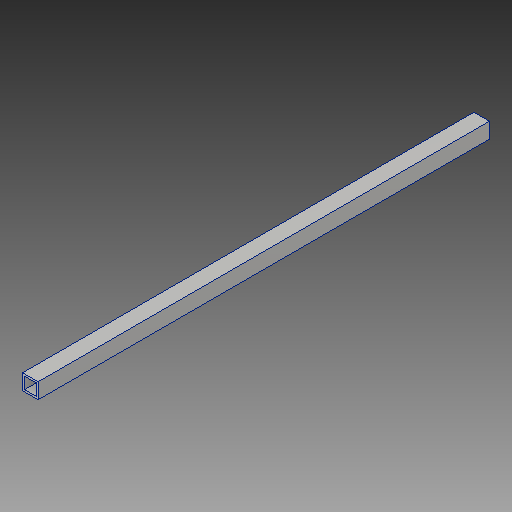
# Autodesk Inventor part: 1by1by31
Saved by Autodesk Inventor 2018 (Build 220112000, 112)
## iProperties
Created: 2018-01-13
Part Number: 1by1by31
Material: Aluminum 6061
Document SubType Name: Modeling
Designer: s-4000369
Density: 2.7 g/cm^3
Appearance: Aluminum - Flat
Mass: 561.359 g
Surface Area: 1315.32 cm^2
Volume: 207.911 cm^3
Author: s-4000369
Autodesk Inventor part; units mm, degrees
ref_plane "YZ Plane" through (0, 0, 0) normal (1, 0, 0) x (0, 1, 0)
ref_plane "XZ Plane" through (0, 0, 0) normal (0, 1, 0) x (-1, 0, 0)
ref_plane "XY Plane" through (0, 0, 0) normal (0, 0, 1) x (1, 0, 0)
sketch "Sketch1" plane through (0, 0, 0) normal (1, 0, 0) x (0, 1, 0)
  line L0 (0, 0) -> (25.4, 0)
  line L1 (25.4, 0) -> (25.4, -787.4)
  line L2 (25.4, -787.4) -> (0, -787.4)
  line L3 (0, -787.4) -> (0, 0)
  dimension "d0" = 787.4
  dimension "d1" = 25.4
  constraints: 8 end point, 2 parallel, 1 horizontal, 1 perpendicular
  measures "d0" distance of L0.end L1.end
  measures "d1" distance of L0.start L0.end
extrude "Extrusion1" add sketch "Sketch1" along normal blind 25.4
sketch "Sketch2" plane through (0, 0, 0) normal (0, 0, 1) x (1, 0, 0)
  line L0 (3.175, 3.175) -> (22.225, 3.175)
  line L1 (22.225, 3.175) -> (22.225, 22.225)
  line L2 (22.225, 22.225) -> (3.175, 22.225)
  line L3 (3.175, 22.225) -> (3.175, 3.175)
  line L4 (0, 25.4) -> (25.4, 25.4) projected
  line L5 (0, 0) -> (0, 25.4) projected
  dimension "d4" = 3.175
  dimension "d5" = 3.175
  dimension "d6" = 19.05
  dimension "d7" = 19.05
  constraints: 8 end point, 2 parallel, 1 horizontal, 1 perpendicular
  measures "d4" distance between parallel lines of L4 L2
  measures "d5" distance between parallel lines of L5 L3
  measures "d6" distance of L0.end L1.end
  measures "d7" distance of L0.start L0.end
extrude "Extrusion2" cut sketch "Sketch2" against normal blind 787.4
sketch "Sketch3" plane through (0, 0, 0) normal (0, 0, 1) x (1, 0, 0)
  line L0 (-24.3318, 33.3766) -> (65.9681, 33.3766)
  line L1 (65.9681, 33.3766) -> (65.9681, -31.7467)
  line L2 (65.9681, -31.7467) -> (-24.3318, -31.7467)
  line L3 (-24.3318, -31.7467) -> (-24.3318, 33.3766)
  point P0 (0, 0)
  constraints: 8 end point, 2 parallel, 1 horizontal, 1 perpendicular
extrude "Extrusion3" cut sketch "Sketch3" against normal blind 50.8
body "Solid1"
